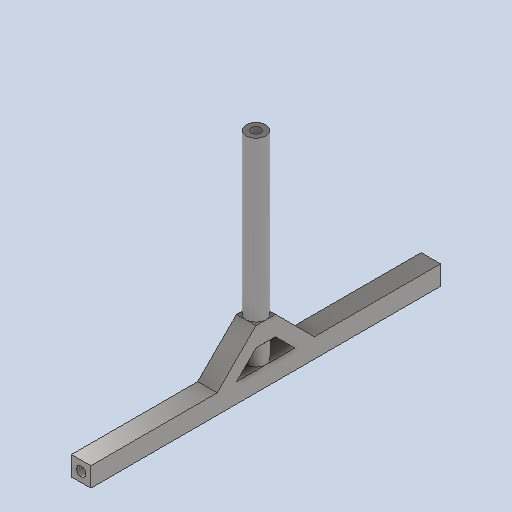
# Autodesk Inventor part: Część L1
Saved by Autodesk Inventor 2022.1 (Build 261234020, 234B)
## iProperties
Created: 2022-05-02
Part Number: Część L1
Material: Stal nierdzewna 440C
Document SubType Name: Modeling
Designer: Kacper Kaczmarski
Density: 7.75 g/cm^3
Appearance: Częściowo polerowany
Mass: 27.3135 g
Surface Area: 31.5175 cm^2
Volume: 3.52432 cm^3
Author: Kacper Kaczmarski
Autodesk Inventor part; units mm, degrees
ref_plane "YZ Plane" through (0, 0, 0) normal (1, 0, 0) x (0, 1, 0)
ref_plane "XZ Plane" through (0, 0, 0) normal (0, 1, 0) x (-1, 0, 0)
ref_plane "XY Plane" through (0, 0, 0) normal (0, 0, 1) x (1, 0, 0)
sketch "Szkic1" plane through (0, 0, 0) normal (0, 1, 0) x (-1, 0, 0)
  circle A0 centre (0, 0) radius 2.5
  dimension "d0" = 5
  constraints: 1 centre point, 1 coincident
  measures "d0" diameter of A0
extrude "Wyciągnięcie proste1" add sketch "Szkic1" along normal blind 48
sketch "Szkic2" plane through (0, 0, 0) normal (0, -1, 0) x (1, 0, 0)
  line L0 (2.5, -45) -> (2.5, 45)
  line L1 (2.5, 45) -> (-2.5, 45)
  line L2 (-2.5, 45) -> (-2.5, -45)
  line L3 (-2.5, -45) -> (2.5, -45)
  line L4 (2.5, -45) -> (-2.5, 45) construction
  line L5 (2.5, 45) -> (-2.5, -45) construction
  point P0 (0, 0)
  dimension "d3" = 90
  constraints: 12 end point, 2 midpoint, 2 parallel, 1 perpendicular, 1 vertical
  measures "d3" distance of L0.start L0.end
extrude "Wyciągnięcie proste2" add sketch "Szkic2" along normal blind 5
sketch "Szkic4" plane through (2.5, 0, -45) normal (0, 0, -1) x (-1, 0, 0)
  line L0 (5, 0) -> (5, -5) projected
  line L1 (5, -2.5) -> (0, -2.5)
  line L2 (0, 0) -> (0, -5) projected
  line L3 (0, -5) -> (5, -5) projected
  line L4 (2.5, -5) -> (2.5, 0)
  point P0 (2.5, -2.5)
  constraints: 4 end point, 4 midpoint, 1 vertical
hole "Otwór2" at (0, -2.5, -45) direction (0, 0, 1) diameter 2.459 depth 8.8 tip angle 118 thread size "M3x0.5" class "6H" standard "ISO Metric profile"
sketch "Szkic5" plane through (-2.5, 0, 45) normal (0, 0, 1) x (1, 0, 0)
  line L0 (0, -5) -> (5, -5) projected
  line L1 (2.5, -5) -> (2.5, 0)
  line L2 (2.5, 0) -> (5, -2.5)
  line L3 (5, 0) -> (5, -5) projected
  line L4 (0, 0) -> (0, -5) projected
  line L5 (0, -2.5) -> (5, -2.5)
  circle A0 centre (2.5, -2.5) radius 1.2295 projected
  constraints: 6 end point, 3 midpoint, 1 coincident, 1 perpendicular, 1 vertical
hole "Otwór3" at (0, -2.5, 45) direction (0, 0, -1) diameter 2.459 depth 8.8 tip angle 118 thread size "M3x0.5" class "6H" standard "ISO Metric profile"
sketch "Szkic7" plane through (2.5, 0, 0) normal (1, 0, 0) x (0, 0, -1)
  line L0 (-45, -5) -> (45, -5) projected
  line L1 (-10, -5) -> (-10, 0)
  line L2 (0, -15.6) -> (0, 58.6) projected
  line L3 (10, -5) -> (10, 0)
  line L4 (10, -2.5) -> (-10, -2.5)
  line L5 (45, 0) -> (0, 0) projected
  line L6 (12.5, -5) -> (7.5, -5)
  line L7 (7.5, -5) -> (7.5, 0)
  line L8 (7.5, 0) -> (12.5, 0)
  line L9 (12.5, 0) -> (12.5, -5)
  line L10 (0, 0) -> (-45, 0) projected
  line L11 (-7.5, -5) -> (-12.5, -5)
  line L12 (-12.5, -5) -> (-12.5, 0)
  line L13 (-12.5, 0) -> (-7.5, 0)
  line L14 (-7.5, 0) -> (-7.5, -5)
  line L15 (2.5, 0) -> (2.5, 48) projected
  line L16 (2.5, 7.5) -> (-2.5498, 7.5)
  line L17 (2.5, 5) -> (-2.5, 5)
  line L18 (-2.5, 5) -> (-2.5, 10)
  line L19 (-2.5, 10) -> (2.5, 10)
  line L20 (2.5, 10) -> (2.5, 5)
  line L21 (12.5, 0) -> (2.5, 10)
  line L22 (7.5, 0) -> (2.5, 5)
  line L23 (-2.5, 5) -> (-7.5, 0)
  line L24 (-12.5, 0) -> (-2.5, 10)
  point P0 (0, -2.5)
  point P1 (0, 7.509)
  dimension "d28" = 10
  dimension "d29" = 5
  dimension "d30" = 5
  dimension "d31" = 5
  dimension "d32" = 5
  constraints: 40 end point, 9 point on line, 7 parallel, 5 perpendicular, 3 horizontal, 2 midpoint, 2 symmetric about line, 1 vertical, 3 other
  measures "d28" distance from line of L4.end L2
  measures "d29" distance of L7.end L8.end
  measures "d30" distance of L12.end L13.end
  measures "d31" distance of L18.end L19.end
  measures "d32" distance of L17.end L18.end
extrude "Wyciągnięcie proste3" add sketch "Szkic7" against normal blind 5 contours L24 L18 L23 L10 | L19 L2 L16 L18 | L16 L2 L17 L18 | L19 L15 L16 L2 | L16 L15 L17 L2 | L21 L5 L22 L15
sketch "Szkic8" plane through (0, 48, 0) normal (0, 1, 0) x (1, 0, 0)
  circle A0 centre (0, 0) radius 2.5
  constraints: 1 centre point, 1 coincident
extrude "Wyciągnięcie proste4" add sketch "Szkic8" along normal blind 3
sketch "Szkic9" plane through (0, 51, 0) normal (0, 1, 0) x (1, 0, 0)
  point P0 (0, 0)
  point P1 (0, 0)
  constraints: 1 coincident
hole "Otwór4" at (0, 51, 0) direction (0, -1, 0) diameter 2.459 depth 8.8 tip angle 118 thread size "M3x0.5" class "6H" standard "ISO Metric profile"
